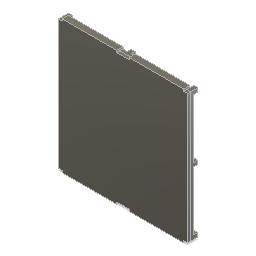
LED Cover v2 (Autodesk Fusion 360 design; units mm, degrees)
Autodesk Fusion 360 part; units mm, degrees
(part 1 of 3)
sketch "Skizze1" plane through (0, 0, 0) normal (0, 0, 1) x (1, 0, 0)
  line L0 (0, 0) -> (161, 0)
  line L1 (161, 0) -> (161, 161)
  line L2 (161, 161) -> (0, 161)
  line L3 (0, 161) -> (0, 0)
  line L4 (0, 0) -> (-2.4, 0) construction
  line L5 (-2.4, 0) -> (-2.4, -2.4) construction
  line L6 (-2.4, -2.4) -> (0, -2.4) construction
  line L7 (0, -2.4) -> (0, 0) construction
  line L8 (-2.4, -2.4) -> (163.4, -2.4)
  line L9 (163.4, -2.4) -> (163.4, 163.4)
  line L10 (163.4, 163.4) -> (-2.4, 163.4)
  line L11 (-2.4, 163.4) -> (-2.4, -2.4)
  dimension "d1" = 161
  dimension "d2" = 161
  dimension "d3" = 2.4
  dimension "d5" = 2.4
  dimension "d6" = 165.8
  dimension "d7" = 165.8
  constraint horizontal L0
  constraint vertical L1
  constraint horizontal L2
  constraint vertical L3
  constraint coincident L0.start L3.end
  constraint horizontal L4
  constraint vertical L5
  constraint horizontal L6
  constraint vertical L7
  constraint horizontal L8
  constraint vertical L9
  constraint horizontal L10
  constraint vertical L11
  measures "d1" distance of L0.start L0.end
  measures "d2" distance of L0.start L2.end
  measures "d3" distance of L5.end L6.end
  measures "d5" distance of L4.end L5.end
  measures "d6" distance of L5.end L8.end
  measures "d7" distance of L5.end L10.end
extrude "Extrusion1" add sketch "Skizze1" against normal blind 4 contours L0 L1 L2 L3 | L8 L9 L10 L11 makes body 1
sketch "Skizze2" plane through (0, 0, -4) normal (0, 0, -1) x (-1, 0, 0)
  line L0 (2.4, -2.4) -> (2.4, 163.4)
  line L1 (2.4, 163.4) -> (-163.4, 163.4)
  line L2 (-163.4, 163.4) -> (-163.4, -2.4)
  line L3 (-163.4, -2.4) -> (2.4, -2.4)
  line L4 (2.4, 163.4) -> (0, 163.4) construction
  line L5 (0, 163.4) -> (0, 161) construction
  line L6 (0, 161) -> (2.4, 161) construction
  line L7 (2.4, 161) -> (2.4, 163.4) construction
  line L8 (0, 161) -> (-35, 161) construction
  line L9 (-35, 161) -> (-35, 131) construction
  line L10 (-35, 131) -> (-35, 111) construction
  line L11 (-35, 111) -> (-35, 91) construction
  line L12 (-35, 91) -> (-35, 71) construction
  line L13 (-35, 71) -> (-35, 51) construction
  line L14 (-35, 51) -> (-35, 31) construction
  circle A0 centre (-35, 121) radius 10
  circle A1 centre (-35, 81) radius 10
  circle A2 centre (-35, 41) radius 10
  line L15 (-25, 121) -> (2.4, 121) construction
  line L16 (2.4, 121) -> (2.4, 116)
  line L17 (2.4, 116) -> (-26.3397, 116)
  line L18 (2.4, 121) -> (2.4, 126) construction
  line L19 (2.4, 126) -> (-26.3397, 126)
  line L20 (2.4, 81) -> (2.4, 76)
  line L21 (2.4, 76) -> (-26.3397, 76)
  line L22 (2.4, 81) -> (2.4, 86)
  line L23 (2.4, 86) -> (-26.3397, 86)
  line L24 (2.4, 41) -> (2.4, 36)
  line L25 (2.4, 36) -> (-26.3397, 36)
  line L26 (2.4, 41) -> (2.4, 46)
  line L27 (2.4, 46) -> (-26.3397, 46)
  line L28 (-25, 121) -> (-35, 121) construction
  line L29 (-35, 31) -> (2.4, 31) construction
  line L30 (-35, 51) -> (2.4, 51) construction
  line L31 (-35, 71) -> (2.4, 71) construction
  line L32 (-35, 91) -> (2.4, 91) construction
  line L33 (-35, 111) -> (2.4, 111) construction
  line L34 (-35, 131) -> (2.4, 131) construction
  line L35 (2.4, 131) -> (-2.6, 131)
  line L36 (-2.6, 131) -> (-2.6, 111)
  line L37 (-2.6, 111) -> (2.4, 111)
  line L38 (2.4, 111) -> (2.4, 131)
  line L39 (2.4, 91) -> (-2.6, 91)
  line L40 (-2.6, 91) -> (-2.6, 71)
  line L41 (-2.6, 71) -> (2.4, 71)
  line L42 (2.4, 71) -> (2.4, 91)
  line L43 (2.4, 51) -> (-2.6, 51)
  line L44 (-2.6, 51) -> (-2.6, 31)
  line L45 (-2.6, 31) -> (2.4, 31)
  line L46 (2.4, 31) -> (2.4, 51)
  line L47 (2.4, -2.4) -> (-2.6, -2.4)
  line L48 (-2.6, -2.4) -> (-2.6, 2.6)
  line L49 (-2.6, 2.6) -> (2.4, 2.6)
  line L50 (2.4, 2.6) -> (2.4, -2.4)
  line L51 (-78, 2.6) -> (-78, -2.4)
  line L52 (-78, -2.4) -> (-83, -2.4)
  line L53 (-83, 2.6) -> (-78, 2.6)
  line L54 (-83, -2.4) -> (-83, 2.6)
  line L55 (-158.4, 2.6) -> (-158.4, -2.4)
  line L56 (-158.4, -2.4) -> (-163.4, -2.4)
  line L57 (-163.4, 2.6) -> (-158.4, 2.6)
  line L58 (-163.4, -2.4) -> (-163.4, 2.6)
  line L59 (2.4, 83) -> (2.4, 78)
  line L60 (2.4, 78) -> (-2.6, 78)
  line L61 (-2.6, 83) -> (2.4, 83)
  line L62 (-2.6, 78) -> (-2.6, 83)
  line L63 (-78, 83) -> (-78, 78)
  line L64 (-78, 78) -> (-83, 78)
  line L65 (-83, 83) -> (-78, 83)
  line L66 (-83, 78) -> (-83, 83)
  line L67 (-158.4, 83) -> (-158.4, 78)
  line L68 (-158.4, 78) -> (-163.4, 78)
  line L69 (-163.4, 83) -> (-158.4, 83)
  line L70 (-163.4, 78) -> (-163.4, 83)
  line L71 (2.4, 163.4) -> (2.4, 158.4)
  line L72 (2.4, 158.4) -> (-2.6, 158.4)
  line L73 (-2.6, 163.4) -> (2.4, 163.4)
  line L74 (-2.6, 158.4) -> (-2.6, 163.4)
  line L75 (-78, 163.4) -> (-78, 158.4)
  line L76 (-78, 158.4) -> (-83, 158.4)
  line L77 (-83, 163.4) -> (-78, 163.4)
  line L78 (-83, 158.4) -> (-83, 163.4)
  line L79 (-158.4, 163.4) -> (-158.4, 158.4)
  line L80 (-158.4, 158.4) -> (-163.4, 158.4)
  line L81 (-163.4, 163.4) -> (-158.4, 163.4)
  line L82 (-163.4, 158.4) -> (-163.4, 163.4)
  circle A3 centre (-35, 121) radius 10.9
  line L83 (-26.3397, 126) -> (-26.3397, 127.8) construction
  line L84 (-26.3397, 127.8) -> (-2.6, 127.8)
  line L85 (-26.3397, 127.8) -> (-27.6679, 127.8)
  line L86 (-26.3397, 114.2) -> (-27.6679, 114.2)
  line L87 (-26.3397, 114.2) -> (-2.6, 114.2)
  line L88 (-26.3397, 74.2) -> (-2.6, 74.2)
  line L89 (-26.3397, 74.2) -> (-27.6679, 74.2)
  line L90 (-26.3397, 87.8) -> (-27.6679, 87.8)
  line L91 (-26.3397, 87.8) -> (-2.6, 87.8)
  circle A4 centre (-35, 81) radius 10.9
  line L92 (-26.3397, 34.2) -> (-2.6, 34.2)
  line L93 (-26.3397, 34.2) -> (-27.6679, 34.2)
  line L94 (-26.3397, 47.8) -> (-27.6679, 47.8)
  line L95 (-26.3397, 47.8) -> (-2.6, 47.8)
  circle A5 centre (-35, 41) radius 10.9
  dimension "d12" = 2.4
  dimension "d13" = 2.4
  dimension "d14" = 35
  dimension "d15" = 30
  dimension "d16" = 20
  dimension "d17" = 20
  dimension "d18" = 20
  dimension "d19" = 20
  dimension "d20" = 20
  dimension "d21" = 20
  dimension "d22" = 20
  dimension "d23" = 20
  dimension "d24" = 5
  dimension "d27" = 0
  dimension "d28" = -80
  dimension "d31" = 5
  dimension "d32" = 5
  dimension "d33" = 5
  dimension "d34" = 5
  dimension "d35" = 5
  dimension "d38" = -160.8
  dimension "d39" = 160.8
  dimension "d74" = 21.8
  dimension "d75" = 1.8
  constraint horizontal L4
  constraint vertical L5
  constraint horizontal L6
  constraint vertical L7
  constraint coincident L0.end L1.start
  constraint perpendicular L5 L8
  constraint perpendicular L8 L9
  constraint parallel L9 L10
  constraint parallel L10 L11
  constraint parallel L11 L12
  constraint parallel L12 L13
  constraint parallel L13 L14
  constraint midpoint L10 A0.centre
  constraint midpoint L12 A1.centre
  constraint coincident L14 A2.centre
  constraint coincident A0 L15.start
  constraint coincident L0 L15.end
  constraint perpendicular L0 L15
  constraint perpendicular L15 L16
  constraint horizontal L17
  constraint coincident A0 L17.end
  constraint symmetric L16.start L15 L18.start
  constraint symmetric L15 L16.end L18.end
  constraint symmetric L15 L17.end L19.end
  constraint midpoint L14 A2.centre
  constraint coincident A0.centre L28.end
  constraint perpendicular L10 L28
  constraint coincident L0 L29.end
  constraint tangent A2 L29
  constraint perpendicular L0 L29
  constraint coincident L0 L30.end
  constraint tangent A2 L30
  constraint perpendicular L0 L30
  constraint coincident L0 L31.end
  constraint tangent A1 L31
  constraint perpendicular L0 L31
  constraint coincident L0 L32.end
  constraint tangent A1 L32
  constraint perpendicular L0 L32
  constraint coincident L0 L33.end
  constraint tangent A0 L33
  constraint perpendicular L0 L33
  constraint coincident L0 L34.end
  constraint tangent A0 L34
  constraint perpendicular L0 L34
  constraint horizontal L35
  constraint vertical L36
  constraint horizontal L37
  constraint vertical L38
  constraint horizontal L39
  constraint vertical L40
  constraint horizontal L41
  constraint vertical L42
  constraint coincident L31 L40.end
  constraint horizontal L43
  constraint vertical L44
  constraint horizontal L45
  constraint vertical L46
  constraint coincident L29 L44.end
  constraint horizontal L47
  constraint vertical L48
  constraint horizontal L49
  constraint vertical L50
  constraint coincident L0.start L3.end
  constraint vertical L83
  constraint horizontal L84
  constraint coincident L36 L84.end
  constraint coincident A0 L85.end
  constraint perpendicular L83 L85
  constraint symmetric L15 L83.end L86.start
  constraint symmetric L15 L84.end L87.end
  constraint symmetric L15 L85.end L86.end
  measures "d12" distance of L0.end L4.end
  measures "d13" distance of L0.end L6.end
  measures "d14" distance of L5.end L8.end
  measures "d15" distance of L8.end L9.end
  measures "d16" distance of L9.end L10.end
  measures "d17" distance of L10.end L11.end
  measures "d18" distance of L11.end L12.end
  measures "d19" distance of L12.end L13.end
  measures "d20" distance of L13.end L14.end
  measures "d24" distance of L15.end L16.end
  measures "d31" distance of L34.end L35.end
  measures "d32" distance of L32.end L39.end
  measures "d33" distance of L30.end L43.end
  measures "d34" distance of L0.start L47.end
  measures "d35" distance of L0.start L49.end
  measures "d75" distance of L19.end L83.end
extrude "Extrusion3" cut sketch "Skizze2" against normal blind 5 contours L0 L24 L25 L26 L27 L44 L46 | L25 L27 L44 A5 | A2 L25 L27 A5 | A2 | L0 L20 L21 L40 L42 L60 | L0 L20 L22 L40 L42 L59 L60 L61 L62 | L21 L23 L40 L62 A4 | A1 L21 L23 A4 | L0 L22 L23 L40 L42 L61 | A1 | L0 L16 L17 L19 L36 L38 | L17 L19 L36 A3 | A0 L17 L19 A3 | A0 bodies 1
extrude "Extrusion4" add sketch "Skizze2" along normal blind 5 contours L0 L3 L47 L48 L49 L50 | L3 L51 L52 L53 L54 | L2 L3 L55 L56 L57 L58 | L2 L67 L68 L69 L70 | L0 L20 L22 L40 L42 L59 L60 L61 L62 | L1 L2 L79 L80 L81 L82 | L1 L75 L76 L77 L78 | L0 L1 L71 L72 L73 L74 | L63 L64 L65 L66 bodies 1 makes body 2 at (-0.7333, 78, -5.6667)
extrude "Extrusion9" add sketch "Skizze2" along normal blind 1 contours L0 L25 L44 L45 L46 | L0 L24 L25 L26 L27 L44 L46 | L25 L44 L92 L93 A5 | L25 L27 L44 A5 | L0 L27 L43 L44 L46 | A2 L25 L93 A5 | A2 L25 L27 A5 | L27 L44 L94 L95 A5 | A2 | A2 L93 L94 A5 | A2 L27 L94 A5 | L0 L21 L40 L41 L42 | L0 L20 L21 L40 L42 L60 | L0 L20 L22 L40 L42 L59 L60 L61 L62 | L21 L40 L88 L89 A4 | L21 L23 L40 L62 A4 | A1 L21 L89 A4 | A1 L21 L23 A4 | L0 L22 L23 L40 L42 L61 | A1 | A1 L89 L90 A4 | L0 L23 L39 L40 L42 | L23 L40 L90 L91 A4 | A1 L23 L90 A4 | L0 L17 L36 L37 L38 | L0 L16 L17 L19 L36 L38 | L17 L36 A3 L86 L87 | L17 L19 L36 A3 | L0 L19 L35 L36 L38 | A0 L17 A3 L86 | A0 L17 L19 A3 | L19 L36 A3 L84 L85 | A0 | A0 A3 L85 L86 | A0 L19 A3 L85 bodies 2 1
sketch "Skizze3" plane through (0, 0, 0) normal (0, 0, 1) x (1, 0, 0)
  line L0 (-2.4, 86) -> (26.3397, 86)
  arc A0 (26.3397, 76) -> (26.3397, 86) centre (35, 81) ccw
  line L1 (26.3397, 76) -> (-2.4, 76)
  line L2 (-2.4, 76) -> (-2.4, 46)
  line L3 (-2.4, 46) -> (26.3397, 46)
  arc A1 (26.3397, 36) -> (26.3397, 46) centre (35, 41) ccw
  line L4 (26.3397, 36) -> (-2.4, 36)
  line L5 (-2.4, 36) -> (-2.4, -2.4)
  line L6 (-2.4, -2.4) -> (163.4, -2.4)
  line L7 (163.4, -2.4) -> (163.4, 163.4)
  line L8 (163.4, 163.4) -> (-2.4, 163.4)
  line L9 (-2.4, 163.4) -> (-2.4, 126)
  line L10 (-2.4, 126) -> (26.3397, 126)
  arc A2 (26.3397, 116) -> (26.3397, 126) centre (35, 121) ccw
  line L11 (26.3397, 116) -> (-2.4, 116)
  line L12 (-2.4, 116) -> (-2.4, 86)
  line L13 (163.4, 163.4) -> (-2.4, 163.4)
  line L14 (-2.4, 163.4) -> (-2.4, -2.4)
  line L15 (-2.4, -2.4) -> (163.4, -2.4)
  line L16 (163.4, -2.4) -> (163.4, 163.4)
  line L17 (-2.4, -2.4) -> (0, -2.4) construction
  line L18 (0, -2.4) -> (0, 0) construction
  line L19 (0, 0) -> (-2.4, 0) construction
  line L20 (-2.4, 0) -> (-2.4, -2.4) construction
  line L21 (0, 0) -> (161, 0)
  line L22 (161, 0) -> (161, 161)
  line L23 (161, 161) -> (0, 161)
  line L24 (0, 161) -> (0, 0)
  line L25 (-2.4, 163.4) -> (72.6, 163.4)
  line L26 (72.6, 163.4) -> (72.6, 165.9)
  line L27 (72.6, 165.9) -> (-2.4, 165.9)
  line L28 (-2.4, 165.9) -> (-2.4, 163.4)
  line L29 (-2.4, 165.9) -> (2.6, 165.9) construction
  line L30 (2.6, 165.9) -> (2.6, 163.4)
  line L31 (2.6, 163.4) -> (2.6, 161)
  line L32 (80.5, 161) -> (80.5, 144.4743) construction
  line L33 (161, 80.5) -> (141.9366, 80.5) construction
  line L34 (163.4, 163.4) -> (88.4, 163.4)
  line L35 (88.4, 163.4) -> (88.4, 165.9)
  line L36 (88.4, 165.9) -> (163.4, 165.9)
  line L37 (163.4, 165.9) -> (163.4, 163.4)
  line L38 (158.4, 163.4) -> (158.4, 161)
  line L39 (158.4, 165.9) -> (158.4, 163.4)
  line L40 (163.4, -2.4) -> (88.4, -2.4)
  line L41 (88.4, -2.4) -> (88.4, -4.9)
  line L42 (88.4, -4.9) -> (163.4, -4.9)
  line L43 (163.4, -4.9) -> (163.4, -2.4)
  line L44 (158.4, -2.4) -> (158.4, 0)
  line L45 (158.4, -4.9) -> (158.4, -2.4)
  line L46 (-2.4, -2.4) -> (72.6, -2.4)
  line L47 (72.6, -2.4) -> (72.6, -4.9)
  line L48 (-2.4, -4.9) -> (-2.4, -2.4)
  line L49 (2.6, -2.4) -> (2.6, 0)
  line L50 (2.6, -4.9) -> (2.6, -2.4)
  line L51 (72.6, -4.9) -> (-2.4, -4.9)
  line L52 (88.4, 163.4) -> (88.4, 161)
  line L53 (72.6, 163.4) -> (72.6, 161)
  line L54 (72.6, -2.4) -> (72.6, 0)
  line L55 (88.4, -2.4) -> (88.4, 0)
  dimension "d42" = 2.4
  dimension "d43" = 2.4
  dimension "d44" = 161
  dimension "d45" = 161
  dimension "d46" = 75
  dimension "d47" = 2.5
  dimension "d48" = 5
  constraint horizontal L13
  constraint vertical L14
  constraint horizontal L15
  constraint vertical L16
  constraint coincident L5.end L6.start
  constraint coincident L7.end L8.start
  constraint horizontal L17
  constraint vertical L18
  constraint horizontal L19
  constraint vertical L20
  constraint horizontal L21
  constraint vertical L22
  constraint horizontal L23
  constraint vertical L24
  constraint coincident L18.end L19.start
  constraint horizontal L25
  constraint vertical L26
  constraint horizontal L27
  constraint vertical L28
  constraint coincident L8.end L9.start
  constraint perpendicular L28 L29
  constraint vertical L30
  constraint coincident L25 L30.end
  constraint coincident L23 L31.end
  constraint perpendicular L23 L31
  constraint midpoint L23 L32.start
  constraint perpendicular L23 L32
  constraint midpoint L22 L33.start
  constraint perpendicular L22 L33
  constraint symmetric L8.end L32 L7.end
  constraint symmetric L25.end L32 L34.end
  constraint symmetric L26.end L32 L35.end
  constraint symmetric L27.end L32 L36.end
  constraint symmetric L29.end L32 L39.start
  constraint symmetric L30.end L32 L38.start
  constraint symmetric L31.end L32 L38.end
  constraint symmetric L8.end L33 L5.end
  constraint symmetric L25.end L33 L46.end
  constraint symmetric L26.end L33 L47.end
  constraint symmetric L27.end L33 L48.start
  constraint symmetric L29.end L33 L50.start
  constraint symmetric L30.end L33 L49.start
  constraint symmetric L31.end L33 L49.end
  constraint symmetric L33 L7.end L6.end
  constraint symmetric L33 L34.end L40.end
  constraint symmetric L33 L35.end L41.end
  constraint symmetric L33 L36.end L42.end
  constraint symmetric L33 L38.start L44.start
  constraint symmetric L33 L38.end L44.end
  constraint symmetric L33 L39.start L45.start
  constraint coincident L23 L52.end
  constraint perpendicular L23 L52
  constraint symmetric L32 L34.end L25.end
  constraint symmetric L32 L52.end L53.end
  constraint symmetric L33 L52.end L55.end
  constraint symmetric L33 L25.end L46.end
  constraint symmetric L33 L53.end L54.end
  measures "d42" distance of L5.end L17.end
  measures "d43" distance of L5.end L19.end
  measures "d44" distance of L18.end L21.end
  measures "d45" distance of L18.end L23.end
  measures "d46" distance of L8.end L25.end
  measures "d47" distance of L8.end L27.end
  measures "d48" distance of L27.end L29.end
extrude "Extrusion5" add sketch "Skizze3" along normal blind 2 separate body contours L0 L11 L12 L14 L24 | L0 L1 L14 L24 | L10 L11 L14 L24 | L1 L2 L3 L14 L24 | L8 L9 L10 L13 L14 L23 L24 L25 L31 | L3 L4 L14 L24 | L4 L5 L6 L14 L15 L21 L24 L46 L49 | L8 L13 L23 L25 L31 L53 | L8 L13 L23 L52 L53 | L6 L15 L21 L46 L49 L54 | L8 L13 L23 L34 L38 L52 | L6 L15 L21 L54 L55 | L6 L7 L8 L13 L15 L16 L21 L22 L23 L34 L38 L40 L44 | L6 L15 L21 L40 L44 L55 makes body 3
extrude "Extrusion6" add sketch "Skizze3" along normal blind 2 from surface at 2 contours L0 L11 L12 L14 L24 | L0 L1 L14 L24 | L0 A0 L1 L3 A1 L4 L10 A2 L11 L21 L22 L23 L24 | L0 A0 L1 L24 | L10 L11 L14 L24 | L1 L2 L3 L14 L24 | L10 A2 L11 L24 | L8 L9 L10 L13 L14 L23 L24 L25 L31 | L3 L4 L14 L24 | L3 A1 L4 L24 | L4 L5 L6 L14 L15 L21 L24 L46 L49 | L8 L13 L23 L25 L31 L53 | L8 L13 L23 L52 L53 | L6 L15 L21 L46 L49 L54 | L8 L13 L23 L34 L38 L52 | L6 L15 L21 L54 L55 | L6 L7 L8 L13 L15 L16 L21 L22 L23 L34 L38 L40 L44 | L6 L15 L21 L40 L44 L55 bodies 3
extrude "Extrusion7" add sketch "Skizze3" along normal up to surface (4 mm away) and the other way up to surface (4 mm away) contours L8 L13 L25 L26 L27 L30 | L6 L15 L46 L47 L50 L51 | L8 L13 L34 L35 L36 L39 | L6 L15 L40 L41 L42 L45 bodies 3
sketch "Skizze4" plane through (0, 0, 2) normal (0, 0, -1) x (-1, 0, 0)
  line L0 (-161, 0) -> (0, 0)
  line L1 (0, 0) -> (0, 161)
  line L2 (0, 161) -> (-161, 161)
  line L3 (-161, 161) -> (-161, 0)
  line L4 (0, 161) -> (-2.4, 161) construction
  line L5 (-2.4, 161) -> (-2.4, 158.6) construction
  line L6 (-2.4, 158.6) -> (0, 158.6) construction
  line L7 (0, 158.6) -> (0, 161) construction
  line L8 (-2.4, 158.6) -> (-158.6, 158.6) construction
  line L9 (-2.4, 158.6) -> (-2.4, 2.4) construction
  line L10 (-2.4, 158.6) -> (-11.4, 158.6)
  line L11 (-11.4, 158.6) -> (-11.4, 152.1)
  line L12 (-11.4, 152.1) -> (-2.4, 152.1)
  line L13 (-2.4, 152.1) -> (-2.4, 158.6)
  line L14 (-2.4, 158.6) -> (-3, 158.6) construction
  line L15 (-3, 158.6) -> (-3, 158) construction
  line L16 (-3, 158) -> (-2.4, 158) construction
  line L17 (-2.4, 158) -> (-2.4, 158.6) construction
  line L18 (-3, 158) -> (-10.8, 158)
  line L19 (-10.8, 158) -> (-10.8, 152.7)
  line L20 (-10.8, 152.7) -> (-3, 152.7)
  line L21 (-3, 152.7) -> (-3, 158)
  line L22 (-20.6533, 152.7) -> (-12.8533, 152.7)
  line L23 (-12.2533, 158.6) -> (-21.2533, 158.6)
  line L24 (-21.2533, 158.6) -> (-21.2533, 152.1)
  line L25 (-12.2533, 152.1) -> (-12.2533, 158.6)
  line L26 (-21.2533, 152.1) -> (-12.2533, 152.1)
  line L27 (-20.6533, 158) -> (-20.6533, 152.7)
  line L28 (-12.8533, 158) -> (-20.6533, 158)
  line L29 (-12.8533, 152.7) -> (-12.8533, 158)
  line L30 (-30.5067, 152.7) -> (-22.7067, 152.7)
  line L31 (-22.1067, 158.6) -> (-31.1067, 158.6)
  line L32 (-31.1067, 158.6) -> (-31.1067, 152.1)
  line L33 (-22.1067, 152.1) -> (-22.1067, 158.6)
  line L34 (-31.1067, 152.1) -> (-22.1067, 152.1)
  line L35 (-30.5067, 158) -> (-30.5067, 152.7)
  line L36 (-22.7067, 158) -> (-30.5067, 158)
  line L37 (-22.7067, 152.7) -> (-22.7067, 158)
  line L38 (-40.36, 152.7) -> (-32.56, 152.7)
  line L39 (-31.96, 158.6) -> (-40.96, 158.6)
  line L40 (-40.96, 158.6) -> (-40.96, 152.1)
  line L41 (-31.96, 152.1) -> (-31.96, 158.6)
  line L42 (-40.96, 152.1) -> (-31.96, 152.1)
  line L43 (-40.36, 158) -> (-40.36, 152.7)
  line L44 (-32.56, 158) -> (-40.36, 158)
  line L45 (-32.56, 152.7) -> (-32.56, 158)
  line L46 (-50.2133, 152.7) -> (-42.4133, 152.7)
  line L47 (-41.8133, 158.6) -> (-50.8133, 158.6)
  line L48 (-50.8133, 158.6) -> (-50.8133, 152.1)
  line L49 (-41.8133, 152.1) -> (-41.8133, 158.6)
  line L50 (-50.8133, 152.1) -> (-41.8133, 152.1)
  line L51 (-50.2133, 158) -> (-50.2133, 152.7)
  line L52 (-42.4133, 158) -> (-50.2133, 158)
  line L53 (-42.4133, 152.7) -> (-42.4133, 158)
  line L54 (-60.0667, 152.7) -> (-52.2667, 152.7)
  line L55 (-51.6667, 158.6) -> (-60.6667, 158.6)
  line L56 (-60.6667, 158.6) -> (-60.6667, 152.1)
  line L57 (-51.6667, 152.1) -> (-51.6667, 158.6)
  line L58 (-60.6667, 152.1) -> (-51.6667, 152.1)
  line L59 (-60.0667, 158) -> (-60.0667, 152.7)
  line L60 (-52.2667, 158) -> (-60.0667, 158)
  line L61 (-52.2667, 152.7) -> (-52.2667, 158)
  line L62 (-69.92, 152.7) -> (-62.12, 152.7)
  line L63 (-61.52, 158.6) -> (-70.52, 158.6)
  line L64 (-70.52, 158.6) -> (-70.52, 152.1)
  line L65 (-61.52, 152.1) -> (-61.52, 158.6)
  line L66 (-70.52, 152.1) -> (-61.52, 152.1)
  line L67 (-69.92, 158) -> (-69.92, 152.7)
  line L68 (-62.12, 158) -> (-69.92, 158)
  line L69 (-62.12, 152.7) -> (-62.12, 158)
  line L70 (-79.7733, 152.7) -> (-71.9733, 152.7)
  line L71 (-71.3733, 158.6) -> (-80.3733, 158.6)
  line L72 (-80.3733, 158.6) -> (-80.3733, 152.1)
  line L73 (-71.3733, 152.1) -> (-71.3733, 158.6)
  line L74 (-80.3733, 152.1) -> (-71.3733, 152.1)
  line L75 (-79.7733, 158) -> (-79.7733, 152.7)
  line L76 (-71.9733, 158) -> (-79.7733, 158)
  line L77 (-71.9733, 152.7) -> (-71.9733, 158)
  line L78 (-89.6267, 152.7) -> (-81.8267, 152.7)
  line L79 (-81.2267, 158.6) -> (-90.2267, 158.6)
  line L80 (-90.2267, 158.6) -> (-90.2267, 152.1)
  line L81 (-81.2267, 152.1) -> (-81.2267, 158.6)
  line L82 (-90.2267, 152.1) -> (-81.2267, 152.1)
  line L83 (-89.6267, 158) -> (-89.6267, 152.7)
  line L84 (-81.8267, 158) -> (-89.6267, 158)
  line L85 (-81.8267, 152.7) -> (-81.8267, 158)
  line L86 (-99.48, 152.7) -> (-91.68, 152.7)
  line L87 (-91.08, 158.6) -> (-100.08, 158.6)
  line L88 (-100.08, 158.6) -> (-100.08, 152.1)
  line L89 (-91.08, 152.1) -> (-91.08, 158.6)
  line L90 (-100.08, 152.1) -> (-91.08, 152.1)
  line L91 (-99.48, 158) -> (-99.48, 152.7)
  line L92 (-91.68, 158) -> (-99.48, 158)
  line L93 (-91.68, 152.7) -> (-91.68, 158)
  line L94 (-109.3333, 152.7) -> (-101.5333, 152.7)
  line L95 (-100.9333, 158.6) -> (-109.9333, 158.6)
  line L96 (-109.9333, 158.6) -> (-109.9333, 152.1)
  line L97 (-100.9333, 152.1) -> (-100.9333, 158.6)
  line L98 (-109.9333, 152.1) -> (-100.9333, 152.1)
  line L99 (-109.3333, 158) -> (-109.3333, 152.7)
  line L100 (-101.5333, 158) -> (-109.3333, 158)
  line L101 (-101.5333, 152.7) -> (-101.5333, 158)
  line L102 (-119.1867, 152.7) -> (-111.3867, 152.7)
  line L103 (-110.7867, 158.6) -> (-119.7867, 158.6)
  line L104 (-119.7867, 158.6) -> (-119.7867, 152.1)
  line L105 (-110.7867, 152.1) -> (-110.7867, 158.6)
  line L106 (-119.7867, 152.1) -> (-110.7867, 152.1)
  line L107 (-119.1867, 158) -> (-119.1867, 152.7)
  line L108 (-111.3867, 158) -> (-119.1867, 158)
  line L109 (-111.3867, 152.7) -> (-111.3867, 158)
  line L110 (-129.04, 152.7) -> (-121.24, 152.7)
  line L111 (-120.64, 158.6) -> (-129.64, 158.6)
  line L112 (-129.64, 158.6) -> (-129.64, 152.1)
  line L113 (-120.64, 152.1) -> (-120.64, 158.6)
  line L114 (-129.64, 152.1) -> (-120.64, 152.1)
  line L115 (-129.04, 158) -> (-129.04, 152.7)
  line L116 (-121.24, 158) -> (-129.04, 158)
  line L117 (-121.24, 152.7) -> (-121.24, 158)
  line L118 (-138.8933, 152.7) -> (-131.0933, 152.7)
  line L119 (-130.4933, 158.6) -> (-139.4933, 158.6)
  line L120 (-139.4933, 158.6) -> (-139.4933, 152.1)
  line L121 (-130.4933, 152.1) -> (-130.4933, 158.6)
  line L122 (-139.4933, 152.1) -> (-130.4933, 152.1)
  line L123 (-138.8933, 158) -> (-138.8933, 152.7)
  line L124 (-131.0933, 158) -> (-138.8933, 158)
  line L125 (-131.0933, 152.7) -> (-131.0933, 158)
  line L126 (-148.7467, 152.7) -> (-140.9467, 152.7)
  line L127 (-140.3467, 158.6) -> (-149.3467, 158.6)
  line L128 (-149.3467, 158.6) -> (-149.3467, 152.1)
  line L129 (-140.3467, 152.1) -> (-140.3467, 158.6)
  line L130 (-149.3467, 152.1) -> (-140.3467, 152.1)
  line L131 (-148.7467, 158) -> (-148.7467, 152.7)
  line L132 (-140.9467, 158) -> (-148.7467, 158)
  line L133 (-140.9467, 152.7) -> (-140.9467, 158)
  line L134 (-158.6, 152.7) -> (-150.8, 152.7)
  line L135 (-150.2, 158.6) -> (-159.2, 158.6)
  line L136 (-159.2, 158.6) -> (-159.2, 152.1)
  line L137 (-150.2, 152.1) -> (-150.2, 158.6)
  line L138 (-159.2, 152.1) -> (-150.2, 152.1)
  line L139 (-158.6, 158) -> (-158.6, 152.7)
  line L140 (-150.8, 158) -> (-158.6, 158)
  line L141 (-150.8, 152.7) -> (-150.8, 158)
  line L142 (-10.8, 142.68) -> (-3, 142.68)
  line L143 (-2.4, 148.58) -> (-11.4, 148.58)
  line L144 (-11.4, 148.58) -> (-11.4, 142.08)
  line L145 (-2.4, 142.08) -> (-2.4, 148.58)
  line L146 (-11.4, 142.08) -> (-2.4, 142.08)
  line L147 (-10.8, 147.98) -> (-10.8, 142.68)
  line L148 (-3, 147.98) -> (-10.8, 147.98)
  line L149 (-3, 142.68) -> (-3, 147.98)
  line L150 (-20.6533, 142.68) -> (-12.8533, 142.68)
  line L151 (-12.2533, 148.58) -> (-21.2533, 148.58)
  line L152 (-21.2533, 148.58) -> (-21.2533, 142.08)
  line L153 (-12.2533, 142.08) -> (-12.2533, 148.58)
  line L154 (-21.2533, 142.08) -> (-12.2533, 142.08)
  line L155 (-20.6533, 147.98) -> (-20.6533, 142.68)
  line L156 (-12.8533, 147.98) -> (-20.6533, 147.98)
  line L157 (-12.8533, 142.68) -> (-12.8533, 147.98)
  line L158 (-30.5067, 142.68) -> (-22.7067, 142.68)
  line L159 (-22.1067, 148.58) -> (-31.1067, 148.58)
  line L160 (-31.1067, 148.58) -> (-31.1067, 142.08)
  line L161 (-22.1067, 142.08) -> (-22.1067, 148.58)
  line L162 (-31.1067, 142.08) -> (-22.1067, 142.08)
  line L163 (-30.5067, 147.98) -> (-30.5067, 142.68)
  line L164 (-22.7067, 147.98) -> (-30.5067, 147.98)
  line L165 (-22.7067, 142.68) -> (-22.7067, 147.98)
  line L166 (-40.36, 142.68) -> (-32.56, 142.68)
  line L167 (-31.96, 148.58) -> (-40.96, 148.58)
  line L168 (-40.96, 148.58) -> (-40.96, 142.08)
  line L169 (-31.96, 142.08) -> (-31.96, 148.58)
  line L170 (-40.96, 142.08) -> (-31.96, 142.08)
  line L171 (-40.36, 147.98) -> (-40.36, 142.68)
  line L172 (-32.56, 147.98) -> (-40.36, 147.98)
  line L173 (-32.56, 142.68) -> (-32.56, 147.98)
  line L174 (-50.2133, 142.68) -> (-42.4133, 142.68)
  line L175 (-41.8133, 148.58) -> (-50.8133, 148.58)
  line L176 (-50.8133, 148.58) -> (-50.8133, 142.08)
  line L177 (-41.8133, 142.08) -> (-41.8133, 148.58)
  line L178 (-50.8133, 142.08) -> (-41.8133, 142.08)
  line L179 (-50.2133, 147.98) -> (-50.2133, 142.68)
  line L180 (-42.4133, 147.98) -> (-50.2133, 147.98)
  line L181 (-42.4133, 142.68) -> (-42.4133, 147.98)
  line L182 (-60.0667, 142.68) -> (-52.2667, 142.68)
  line L183 (-51.6667, 148.58) -> (-60.6667, 148.58)
  line L184 (-60.6667, 148.58) -> (-60.6667, 142.08)
  line L185 (-51.6667, 142.08) -> (-51.6667, 148.58)
  line L186 (-60.6667, 142.08) -> (-51.6667, 142.08)
  line L187 (-60.0667, 147.98) -> (-60.0667, 142.68)
  line L188 (-52.2667, 147.98) -> (-60.0667, 147.98)
  line L189 (-52.2667, 142.68) -> (-52.2667, 147.98)
  line L190 (-69.92, 142.68) -> (-62.12, 142.68)
  line L191 (-61.52, 148.58) -> (-70.52, 148.58)
  line L192 (-70.52, 148.58) -> (-70.52, 142.08)
  line L193 (-61.52, 142.08) -> (-61.52, 148.58)
  line L194 (-70.52, 142.08) -> (-61.52, 142.08)
  line L195 (-69.92, 147.98) -> (-69.92, 142.68)
  line L196 (-62.12, 147.98) -> (-69.92, 147.98)
  line L197 (-62.12, 142.68) -> (-62.12, 147.98)
  line L198 (-79.7733, 142.68) -> (-71.9733, 142.68)
  line L199 (-71.3733, 148.58) -> (-80.3733, 148.58)
  line L200 (-80.3733, 148.58) -> (-80.3733, 142.08)
  line L201 (-71.3733, 142.08) -> (-71.3733, 148.58)
  line L202 (-80.3733, 142.08) -> (-71.3733, 142.08)
  line L203 (-79.7733, 147.98) -> (-79.7733, 142.68)
  line L204 (-71.9733, 147.98) -> (-79.7733, 147.98)
  line L205 (-71.9733, 142.68) -> (-71.9733, 147.98)
  line L206 (-89.6267, 142.68) -> (-81.8267, 142.68)
  line L207 (-81.2267, 148.58) -> (-90.2267, 148.58)
  line L208 (-90.2267, 148.58) -> (-90.2267, 142.08)
  line L209 (-81.2267, 142.08) -> (-81.2267, 148.58)
  line L210 (-90.2267, 142.08) -> (-81.2267, 142.08)
  line L211 (-89.6267, 147.98) -> (-89.6267, 142.68)
  line L212 (-81.8267, 147.98) -> (-89.6267, 147.98)
  line L213 (-81.8267, 142.68) -> (-81.8267, 147.98)
  line L214 (-99.48, 142.68) -> (-91.68, 142.68)
  line L215 (-91.08, 148.58) -> (-100.08, 148.58)
  line L216 (-100.08, 148.58) -> (-100.08, 142.08)
  line L217 (-91.08, 142.08) -> (-91.08, 148.58)
  line L218 (-100.08, 142.08) -> (-91.08, 142.08)
  line L219 (-99.48, 147.98) -> (-99.48, 142.68)
  line L220 (-91.68, 147.98) -> (-99.48, 147.98)
  line L221 (-91.68, 142.68) -> (-91.68, 147.98)
  line L222 (-109.3333, 142.68) -> (-101.5333, 142.68)
  line L223 (-100.9333, 148.58) -> (-109.9333, 148.58)
  line L224 (-109.9333, 148.58) -> (-109.9333, 142.08)
  line L225 (-100.9333, 142.08) -> (-100.9333, 148.58)
  line L226 (-109.9333, 142.08) -> (-100.9333, 142.08)
  line L227 (-109.3333, 147.98) -> (-109.3333, 142.68)
  line L228 (-101.5333, 147.98) -> (-109.3333, 147.98)
  line L229 (-101.5333, 142.68) -> (-101.5333, 147.98)
  line L230 (-119.1867, 142.68) -> (-111.3867, 142.68)
  line L231 (-110.7867, 148.58) -> (-119.7867, 148.58)
  line L232 (-119.7867, 148.58) -> (-119.7867, 142.08)
  line L233 (-110.7867, 142.08) -> (-110.7867, 148.58)
  line L234 (-119.7867, 142.08) -> (-110.7867, 142.08)
  line L235 (-119.1867, 147.98) -> (-119.1867, 142.68)
  line L236 (-111.3867, 147.98) -> (-119.1867, 147.98)
  line L237 (-111.3867, 142.68) -> (-111.3867, 147.98)
  line L238 (-129.04, 142.68) -> (-121.24, 142.68)
  line L239 (-120.64, 148.58) -> (-129.64, 148.58)
  line L240 (-129.64, 148.58) -> (-129.64, 142.08)
  line L241 (-120.64, 142.08) -> (-120.64, 148.58)
  line L242 (-129.64, 142.08) -> (-120.64, 142.08)
  line L243 (-129.04, 147.98) -> (-129.04, 142.68)
  line L244 (-121.24, 147.98) -> (-129.04, 147.98)
  line L245 (-121.24, 142.68) -> (-121.24, 147.98)
  line L246 (-138.8933, 142.68) -> (-131.0933, 142.68)
  line L247 (-130.4933, 148.58) -> (-139.4933, 148.58)
  line L248 (-139.4933, 148.58) -> (-139.4933, 142.08)
  line L249 (-130.4933, 142.08) -> (-130.4933, 148.58)
  line L250 (-139.4933, 142.08) -> (-130.4933, 142.08)
  line L251 (-138.8933, 147.98) -> (-138.8933, 142.68)
  line L252 (-131.0933, 147.98) -> (-138.8933, 147.98)
  line L253 (-131.0933, 142.68) -> (-131.0933, 147.98)
  line L254 (-148.7467, 142.68) -> (-140.9467, 142.68)
  line L255 (-140.3467, 148.58) -> (-149.3467, 148.58)
  line L256 (-149.3467, 148.58) -> (-149.3467, 142.08)
  line L257 (-140.3467, 142.08) -> (-140.3467, 148.58)
  line L258 (-149.3467, 142.08) -> (-140.3467, 142.08)
  line L259 (-148.7467, 147.98) -> (-148.7467, 142.68)
  line L260 (-140.9467, 147.98) -> (-148.7467, 147.98)
  line L261 (-140.9467, 142.68) -> (-140.9467, 147.98)
  line L262 (-158.6, 142.68) -> (-150.8, 142.68)
  line L263 (-150.2, 148.58) -> (-159.2, 148.58)
  line L264 (-159.2, 148.58) -> (-159.2, 142.08)
  line L265 (-150.2, 142.08) -> (-150.2, 148.58)
  line L266 (-159.2, 142.08) -> (-150.2, 142.08)
  line L267 (-158.6, 147.98) -> (-158.6, 142.68)
  line L268 (-150.8, 147.98) -> (-158.6, 147.98)
  line L269 (-150.8, 142.68) -> (-150.8, 147.98)
  line L270 (-10.8, 132.66) -> (-3, 132.66)
  line L271 (-2.4, 138.56) -> (-11.4, 138.56)
  line L272 (-11.4, 138.56) -> (-11.4, 132.06)
  line L273 (-2.4, 132.06) -> (-2.4, 138.56)
  line L274 (-11.4, 132.06) -> (-2.4, 132.06)
  line L275 (-10.8, 137.96) -> (-10.8, 132.66)
  line L276 (-3, 137.96) -> (-10.8, 137.96)
  line L277 (-3, 132.66) -> (-3, 137.96)
  line L278 (-20.6533, 132.66) -> (-12.8533, 132.66)
  line L279 (-12.2533, 138.56) -> (-21.2533, 138.56)
  line L280 (-21.2533, 138.56) -> (-21.2533, 132.06)
  line L281 (-12.2533, 132.06) -> (-12.2533, 138.56)
  line L282 (-21.2533, 132.06) -> (-12.2533, 132.06)
  line L283 (-20.6533, 137.96) -> (-20.6533, 132.66)
  line L284 (-12.8533, 137.96) -> (-20.6533, 137.96)
  line L285 (-12.8533, 132.66) -> (-12.8533, 137.96)
  line L286 (-30.5067, 132.66) -> (-22.7067, 132.66)
  line L287 (-22.1067, 138.56) -> (-31.1067, 138.56)
  line L288 (-31.1067, 138.56) -> (-31.1067, 132.06)
  line L289 (-22.1067, 132.06) -> (-22.1067, 138.56)
  line L290 (-31.1067, 132.06) -> (-22.1067, 132.06)
  line L291 (-30.5067, 137.96) -> (-30.5067, 132.66)
  line L292 (-22.7067, 137.96) -> (-30.5067, 137.96)
  line L293 (-22.7067, 132.66) -> (-22.7067, 137.96)
  line L294 (-40.36, 132.66) -> (-32.56, 132.66)
  line L295 (-31.96, 138.56) -> (-40.96, 138.56)
  line L296 (-40.96, 138.56) -> (-40.96, 132.06)
  line L297 (-31.96, 132.06) -> (-31.96, 138.56)
  line L298 (-40.96, 132.06) -> (-31.96, 132.06)
  line L299 (-40.36, 137.96) -> (-40.36, 132.66)
  line L300 (-32.56, 137.96) -> (-40.36, 137.96)
  line L301 (-32.56, 132.66) -> (-32.56, 137.96)
  line L302 (-50.2133, 132.66) -> (-42.4133, 132.66)
  line L303 (-41.8133, 138.56) -> (-50.8133, 138.56)
  line L304 (-50.8133, 138.56) -> (-50.8133, 132.06)
  line L305 (-41.8133, 132.06) -> (-41.8133, 138.56)
  line L306 (-50.8133, 132.06) -> (-41.8133, 132.06)
  line L307 (-50.2133, 137.96) -> (-50.2133, 132.66)
  line L308 (-42.4133, 137.96) -> (-50.2133, 137.96)
  line L309 (-42.4133, 132.66) -> (-42.4133, 137.96)
  line L310 (-60.0667, 132.66) -> (-52.2667, 132.66)
  line L311 (-51.6667, 138.56) -> (-60.6667, 138.56)
  line L312 (-60.6667, 138.56) -> (-60.6667, 132.06)
  line L313 (-51.6667, 132.06) -> (-51.6667, 138.56)
  line L314 (-60.6667, 132.06) -> (-51.6667, 132.06)
  line L315 (-60.0667, 137.96) -> (-60.0667, 132.66)
  line L316 (-52.2667, 137.96) -> (-60.0667, 137.96)
  line L317 (-52.2667, 132.66) -> (-52.2667, 137.96)
  line L318 (-69.92, 132.66) -> (-62.12, 132.66)
  line L319 (-61.52, 138.56) -> (-70.52, 138.56)
  line L320 (-70.52, 138.56) -> (-70.52, 132.06)
  line L321 (-61.52, 132.06) -> (-61.52, 138.56)
  line L322 (-70.52, 132.06) -> (-61.52, 132.06)
  line L323 (-69.92, 137.96) -> (-69.92, 132.66)
  line L324 (-62.12, 137.96) -> (-69.92, 137.96)
  line L325 (-62.12, 132.66) -> (-62.12, 137.96)
  line L326 (-79.7733, 132.66) -> (-71.9733, 132.66)
  line L327 (-71.3733, 138.56) -> (-80.3733, 138.56)
  line L328 (-80.3733, 138.56) -> (-80.3733, 132.06)
  line L329 (-71.3733, 132.06) -> (-71.3733, 138.56)
  line L330 (-80.3733, 132.06) -> (-71.3733, 132.06)
  line L331 (-79.7733, 137.96) -> (-79.7733, 132.66)
  line L332 (-71.9733, 137.96) -> (-79.7733, 137.96)
  line L333 (-71.9733, 132.66) -> (-71.9733, 137.96)
  line L334 (-89.6267, 132.66) -> (-81.8267, 132.66)
  line L335 (-81.2267, 138.56) -> (-90.2267, 138.56)
  line L336 (-90.2267, 138.56) -> (-90.2267, 132.06)
  line L337 (-81.2267, 132.06) -> (-81.2267, 138.56)
  line L338 (-90.2267, 132.06) -> (-81.2267, 132.06)
  line L339 (-89.6267, 137.96) -> (-89.6267, 132.66)
  line L340 (-81.8267, 137.96) -> (-89.6267, 137.96)
  line L341 (-81.8267, 132.66) -> (-81.8267, 137.96)
  line L342 (-99.48, 132.66) -> (-91.68, 132.66)
  line L343 (-91.08, 138.56) -> (-100.08, 138.56)
  line L344 (-100.08, 138.56) -> (-100.08, 132.06)
  line L345 (-91.08, 132.06) -> (-91.08, 138.56)
  line L346 (-100.08, 132.06) -> (-91.08, 132.06)
  line L347 (-99.48, 137.96) -> (-99.48, 132.66)
  line L348 (-91.68, 137.96) -> (-99.48, 137.96)
  line L349 (-91.68, 132.66) -> (-91.68, 137.96)
  line L350 (-109.3333, 132.66) -> (-101.5333, 132.66)
  line L351 (-100.9333, 138.56) -> (-109.9333, 138.56)
  line L352 (-109.9333, 138.56) -> (-109.9333, 132.06)
  line L353 (-100.9333, 132.06) -> (-100.9333, 138.56)
  line L354 (-109.9333, 132.06) -> (-100.9333, 132.06)
  line L355 (-109.3333, 137.96) -> (-109.3333, 132.66)
  line L356 (-101.5333, 137.96) -> (-109.3333, 137.96)
  line L357 (-101.5333, 132.66) -> (-101.5333, 137.96)
  line L358 (-119.1867, 132.66) -> (-111.3867, 132.66)
  line L359 (-110.7867, 138.56) -> (-119.7867, 138.56)
  line L360 (-119.7867, 138.56) -> (-119.7867, 132.06)
  line L361 (-110.7867, 132.06) -> (-110.7867, 138.56)
  line L362 (-119.7867, 132.06) -> (-110.7867, 132.06)
  line L363 (-119.1867, 137.96) -> (-119.1867, 132.66)
  line L364 (-111.3867, 137.96) -> (-119.1867, 137.96)
  line L365 (-111.3867, 132.66) -> (-111.3867, 137.96)
  line L366 (-129.04, 132.66) -> (-121.24, 132.66)
  line L367 (-120.64, 138.56) -> (-129.64, 138.56)
  line L368 (-129.64, 138.56) -> (-129.64, 132.06)
  line L369 (-120.64, 132.06) -> (-120.64, 138.56)
  line L370 (-129.64, 132.06) -> (-120.64, 132.06)
  line L371 (-129.04, 137.96) -> (-129.04, 132.66)
  line L372 (-121.24, 137.96) -> (-129.04, 137.96)
  line L373 (-121.24, 132.66) -> (-121.24, 137.96)
  line L374 (-138.8933, 132.66) -> (-131.0933, 132.66)
  line L375 (-130.4933, 138.56) -> (-139.4933, 138.56)
  line L376 (-139.4933, 138.56) -> (-139.4933, 132.06)
  line L377 (-130.4933, 132.06) -> (-130.4933, 138.56)
  line L378 (-139.4933, 132.06) -> (-130.4933, 132.06)
  line L379 (-138.8933, 137.96) -> (-138.8933, 132.66)
  line L380 (-131.0933, 137.96) -> (-138.8933, 137.96)
  line L381 (-131.0933, 132.66) -> (-131.0933, 137.96)
  line L382 (-148.7467, 132.66) -> (-140.9467, 132.66)
  line L383 (-140.3467, 138.56) -> (-149.3467, 138.56)
  line L384 (-149.3467, 138.56) -> (-149.3467, 132.06)
  line L385 (-140.3467, 132.06) -> (-140.3467, 138.56)
  line L386 (-149.3467, 132.06) -> (-140.3467, 132.06)
  line L387 (-148.7467, 137.96) -> (-148.7467, 132.66)
  line L388 (-140.9467, 137.96) -> (-148.7467, 137.96)
  line L389 (-140.9467, 132.66) -> (-140.9467, 137.96)
  line L390 (-158.6, 132.66) -> (-150.8, 132.66)
  line L391 (-150.2, 138.56) -> (-159.2, 138.56)
  line L392 (-159.2, 138.56) -> (-159.2, 132.06)
  line L393 (-150.2, 132.06) -> (-150.2, 138.56)
  line L394 (-159.2, 132.06) -> (-150.2, 132.06)
  line L395 (-158.6, 137.96) -> (-158.6, 132.66)
  line L396 (-150.8, 137.96) -> (-158.6, 137.96)
  line L397 (-150.8, 132.66) -> (-150.8, 137.96)
  line L398 (-10.8, 122.64) -> (-3, 122.64)
  line L399 (-2.4, 128.54) -> (-11.4, 128.54)
  line L400 (-11.4, 128.54) -> (-11.4, 122.04)
  line L401 (-2.4, 122.04) -> (-2.4, 128.54)
  line L402 (-11.4, 122.04) -> (-2.4, 122.04)
  line L403 (-10.8, 127.94) -> (-10.8, 122.64)
  line L404 (-3, 127.94) -> (-10.8, 127.94)
  line L405 (-3, 122.64) -> (-3, 127.94)
  line L406 (-20.6533, 122.64) -> (-12.8533, 122.64)
  line L407 (-12.2533, 128.54) -> (-21.2533, 128.54)
  line L408 (-21.2533, 128.54) -> (-21.2533, 122.04)
  line L409 (-12.2533, 122.04) -> (-12.2533, 128.54)
  line L410 (-21.2533, 122.04) -> (-12.2533, 122.04)
  line L411 (-20.6533, 127.94) -> (-20.6533, 122.64)
  line L412 (-12.8533, 127.94) -> (-20.6533, 127.94)
  line L413 (-12.8533, 122.64) -> (-12.8533, 127.94)
  line L414 (-30.5067, 122.64) -> (-22.7067, 122.64)
  line L415 (-22.1067, 128.54) -> (-31.1067, 128.54)
  line L416 (-31.1067, 128.54) -> (-31.1067, 122.04)
  line L417 (-22.1067, 122.04) -> (-22.1067, 128.54)
  line L418 (-31.1067, 122.04) -> (-22.1067, 122.04)
  line L419 (-30.5067, 127.94) -> (-30.5067, 122.64)
  line L420 (-22.7067, 127.94) -> (-30.5067, 127.94)
  line L421 (-22.7067, 122.64) -> (-22.7067, 127.94)
  line L422 (-40.36, 122.64) -> (-32.56, 122.64)
  line L423 (-31.96, 128.54) -> (-40.96, 128.54)
  line L424 (-40.96, 128.54) -> (-40.96, 122.04)
  line L425 (-31.96, 122.04) -> (-31.96, 128.54)
  line L426 (-40.96, 122.04) -> (-31.96, 122.04)
  line L427 (-40.36, 127.94) -> (-40.36, 122.64)
  line L428 (-32.56, 127.94) -> (-40.36, 127.94)
  line L429 (-32.56, 122.64) -> (-32.56, 127.94)
  line L430 (-50.2133, 122.64) -> (-42.4133, 122.64)
  line L431 (-41.8133, 128.54) -> (-50.8133, 128.54)
  line L432 (-50.8133, 128.54) -> (-50.8133, 122.04)
  line L433 (-41.8133, 122.04) -> (-41.8133, 128.54)
  line L434 (-50.8133, 122.04) -> (-41.8133, 122.04)
  line L435 (-50.2133, 127.94) -> (-50.2133, 122.64)
  line L436 (-42.4133, 127.94) -> (-50.2133, 127.94)
  line L437 (-42.4133, 122.64) -> (-42.4133, 127.94)
  line L438 (-60.0667, 122.64) -> (-52.2667, 122.64)
  line L439 (-51.6667, 128.54) -> (-60.6667, 128.54)
  line L440 (-60.6667, 128.54) -> (-60.6667, 122.04)
  line L441 (-51.6667, 122.04) -> (-51.6667, 128.54)
  line L442 (-60.6667, 122.04) -> (-51.6667, 122.04)
  line L443 (-60.0667, 127.94) -> (-60.0667, 122.64)
  line L444 (-52.2667, 127.94) -> (-60.0667, 127.94)
  line L445 (-52.2667, 122.64) -> (-52.2667, 127.94)
  line L446 (-69.92, 122.64) -> (-62.12, 122.64)
  line L447 (-61.52, 128.54) -> (-70.52, 128.54)
  line L448 (-70.52, 128.54) -> (-70.52, 122.04)
  line L449 (-61.52, 122.04) -> (-61.52, 128.54)
  line L450 (-70.52, 122.04) -> (-61.52, 122.04)
  line L451 (-69.92, 127.94) -> (-69.92, 122.64)
  line L452 (-62.12, 127.94) -> (-69.92, 127.94)
  line L453 (-62.12, 122.64) -> (-62.12, 127.94)
  line L454 (-79.7733, 122.64) -> (-71.9733, 122.64)
  line L455 (-71.3733, 128.54) -> (-80.3733, 128.54)
  line L456 (-80.3733, 128.54) -> (-80.3733, 122.04)
  line L457 (-71.3733, 122.04) -> (-71.3733, 128.54)
  line L458 (-80.3733, 122.04) -> (-71.3733, 122.04)
  line L459 (-79.7733, 127.94) -> (-79.7733, 122.64)
  line L460 (-71.9733, 127.94) -> (-79.7733, 127.94)
  line L461 (-71.9733, 122.64) -> (-71.9733, 127.94)
  line L462 (-89.6267, 122.64) -> (-81.8267, 122.64)
  line L463 (-81.2267, 128.54) -> (-90.2267, 128.54)
  line L464 (-90.2267, 128.54) -> (-90.2267, 122.04)
  line L465 (-81.2267, 122.04) -> (-81.2267, 128.54)
  line L466 (-90.2267, 122.04) -> (-81.2267, 122.04)
  line L467 (-89.6267, 127.94) -> (-89.6267, 122.64)
  line L468 (-81.8267, 127.94) -> (-89.6267, 127.94)
  line L469 (-81.8267, 122.64) -> (-81.8267, 127.94)
  line L470 (-99.48, 122.64) -> (-91.68, 122.64)
  line L471 (-91.08, 128.54) -> (-100.08, 128.54)
  line L472 (-100.08, 128.54) -> (-100.08, 122.04)
  line L473 (-91.08, 122.04) -> (-91.08, 128.54)
  line L474 (-100.08, 122.04) -> (-91.08, 122.04)
  line L475 (-99.48, 127.94) -> (-99.48, 122.64)
  line L476 (-91.68, 127.94) -> (-99.48, 127.94)
  line L477 (-91.68, 122.64) -> (-91.68, 127.94)
  line L478 (-109.3333, 122.64) -> (-101.5333, 122.64)
  line L479 (-100.9333, 128.54) -> (-109.9333, 128.54)
  line L480 (-109.9333, 128.54) -> (-109.9333, 122.04)
  line L481 (-100.9333, 122.04) -> (-100.9333, 128.54)
  line L482 (-109.9333, 122.04) -> (-100.9333, 122.04)
  line L483 (-109.3333, 127.94) -> (-109.3333, 122.64)
  line L484 (-101.5333, 127.94) -> (-109.3333, 127.94)
  line L485 (-101.5333, 122.64) -> (-101.5333, 127.94)
  line L486 (-119.1867, 122.64) -> (-111.3867, 122.64)
  line L487 (-110.7867, 128.54) -> (-119.7867, 128.54)
  line L488 (-119.7867, 128.54) -> (-119.7867, 122.04)
  line L489 (-110.7867, 122.04) -> (-110.7867, 128.54)
  line L490 (-119.7867, 122.04) -> (-110.7867, 122.04)
  line L491 (-119.1867, 127.94) -> (-119.1867, 122.64)
  line L492 (-111.3867, 127.94) -> (-119.1867, 127.94)
  line L493 (-111.3867, 122.64) -> (-111.3867, 127.94)
  line L494 (-129.04, 122.64) -> (-121.24, 122.64)
  line L495 (-120.64, 128.54) -> (-129.64, 128.54)
  line L496 (-129.64, 128.54) -> (-129.64, 122.04)
  line L497 (-120.64, 122.04) -> (-120.64, 128.54)
  line L498 (-129.64, 122.04) -> (-120.64, 122.04)
  line L499 (-129.04, 127.94) -> (-129.04, 122.64)
  line L500 (-121.24, 127.94) -> (-129.04, 127.94)
  line L501 (-121.24, 122.64) -> (-121.24, 127.94)
  line L502 (-138.8933, 122.64) -> (-131.0933, 122.64)
  line L503 (-130.4933, 128.54) -> (-139.4933, 128.54)
  line L504 (-139.4933, 128.54) -> (-139.4933, 122.04)
  line L505 (-130.4933, 122.04) -> (-130.4933, 128.54)
  line L506 (-139.4933, 122.04) -> (-130.4933, 122.04)
  line L507 (-138.8933, 127.94) -> (-138.8933, 122.64)
  line L508 (-131.0933, 127.94) -> (-138.8933, 127.94)
  line L509 (-131.0933, 122.64) -> (-131.0933, 127.94)
  line L510 (-148.7467, 122.64) -> (-140.9467, 122.64)
  line L511 (-140.3467, 128.54) -> (-149.3467, 128.54)
  line L512 (-149.3467, 128.54) -> (-149.3467, 122.04)
  line L513 (-140.3467, 122.04) -> (-140.3467, 128.54)
  line L514 (-149.3467, 122.04) -> (-140.3467, 122.04)
  line L515 (-148.7467, 127.94) -> (-148.7467, 122.64)
  line L516 (-140.9467, 127.94) -> (-148.7467, 127.94)
  line L517 (-140.9467, 122.64) -> (-140.9467, 127.94)
  line L518 (-158.6, 122.64) -> (-150.8, 122.64)
  line L519 (-150.2, 128.54) -> (-159.2, 128.54)
  line L520 (-159.2, 128.54) -> (-159.2, 122.04)
  line L521 (-150.2, 122.04) -> (-150.2, 128.54)
  line L522 (-159.2, 122.04) -> (-150.2, 122.04)
  line L523 (-158.6, 127.94) -> (-158.6, 122.64)
  line L524 (-150.8, 127.94) -> (-158.6, 127.94)
  line L525 (-150.8, 122.64) -> (-150.8, 127.94)
  line L526 (-10.8, 112.62) -> (-3, 112.62)
  line L527 (-2.4, 118.52) -> (-11.4, 118.52)
  line L528 (-11.4, 118.52) -> (-11.4, 112.02)
  line L529 (-2.4, 112.02) -> (-2.4, 118.52)
  line L530 (-11.4, 112.02) -> (-2.4, 112.02)
  line L531 (-10.8, 117.92) -> (-10.8, 112.62)
  line L532 (-3, 117.92) -> (-10.8, 117.92)
  line L533 (-3, 112.62) -> (-3, 117.92)
  line L534 (-20.6533, 112.62) -> (-12.8533, 112.62)
  line L535 (-12.2533, 118.52) -> (-21.2533, 118.52)
  line L536 (-21.2533, 118.52) -> (-21.2533, 112.02)
  line L537 (-12.2533, 112.02) -> (-12.2533, 118.52)
  line L538 (-21.2533, 112.02) -> (-12.2533, 112.02)
  line L539 (-20.6533, 117.92) -> (-20.6533, 112.62)
  line L540 (-12.8533, 117.92) -> (-20.6533, 117.92)
  line L541 (-12.8533, 112.62) -> (-12.8533, 117.92)
  line L542 (-30.5067, 112.62) -> (-22.7067, 112.62)
  line L543 (-22.1067, 118.52) -> (-31.1067, 118.52)
  line L544 (-31.1067, 118.52) -> (-31.1067, 112.02)
  line L545 (-22.1067, 112.02) -> (-22.1067, 118.52)
  line L546 (-31.1067, 112.02) -> (-22.1067, 112.02)
  line L547 (-30.5067, 117.92) -> (-30.5067, 112.62)
  line L548 (-22.7067, 117.92) -> (-30.5067, 117.92)
  line L549 (-22.7067, 112.62) -> (-22.7067, 117.92)
  line L550 (-40.36, 112.62) -> (-32.56, 112.62)
  line L551 (-31.96, 118.52) -> (-40.96, 118.52)
  line L552 (-40.96, 118.52) -> (-40.96, 112.02)
  line L553 (-31.96, 112.02) -> (-31.96, 118.52)
  line L554 (-40.96, 112.02) -> (-31.96, 112.02)
  line L555 (-40.36, 117.92) -> (-40.36, 112.62)
  line L556 (-32.56, 117.92) -> (-40.36, 117.92)
  line L557 (-32.56, 112.62) -> (-32.56, 117.92)
  line L558 (-50.2133, 112.62) -> (-42.4133, 112.62)
  line L559 (-41.8133, 118.52) -> (-50.8133, 118.52)
  line L560 (-50.8133, 118.52) -> (-50.8133, 112.02)
  line L561 (-41.8133, 112.02) -> (-41.8133, 118.52)
  line L562 (-50.8133, 112.02) -> (-41.8133, 112.02)
  line L563 (-50.2133, 117.92) -> (-50.2133, 112.62)
  line L564 (-42.4133, 117.92) -> (-50.2133, 117.92)
  line L565 (-42.4133, 112.62) -> (-42.4133, 117.92)
  line L566 (-60.0667, 112.62) -> (-52.2667, 112.62)
  line L567 (-51.6667, 118.52) -> (-60.6667, 118.52)
  line L568 (-60.6667, 118.52) -> (-60.6667, 112.02)
  line L569 (-51.6667, 112.02) -> (-51.6667, 118.52)
  line L570 (-60.6667, 112.02) -> (-51.6667, 112.02)
  line L571 (-60.0667, 117.92) -> (-60.0667, 112.62)
  line L572 (-52.2667, 117.92) -> (-60.0667, 117.92)
  line L573 (-52.2667, 112.62) -> (-52.2667, 117.92)
  line L574 (-69.92, 112.62) -> (-62.12, 112.62)
  line L575 (-61.52, 118.52) -> (-70.52, 118.52)
  line L576 (-70.52, 118.52) -> (-70.52, 112.02)
  line L577 (-61.52, 112.02) -> (-61.52, 118.52)
  line L578 (-70.52, 112.02) -> (-61.52, 112.02)
  line L579 (-69.92, 117.92) -> (-69.92, 112.62)
  line L580 (-62.12, 117.92) -> (-69.92, 117.92)
  line L581 (-62.12, 112.62) -> (-62.12, 117.92)
  line L582 (-79.7733, 112.62) -> (-71.9733, 112.62)
  line L583 (-71.3733, 118.52) -> (-80.3733, 118.52)
  line L584 (-80.3733, 118.52) -> (-80.3733, 112.02)
  line L585 (-71.3733, 112.02) -> (-71.3733, 118.52)
  line L586 (-80.3733, 112.02) -> (-71.3733, 112.02)
  line L587 (-79.7733, 117.92) -> (-79.7733, 112.62)
  line L588 (-71.9733, 117.92) -> (-79.7733, 117.92)
  line L589 (-71.9733, 112.62) -> (-71.9733, 117.92)
  line L590 (-89.6267, 112.62) -> (-81.8267, 112.62)
  line L591 (-81.2267, 118.52) -> (-90.2267, 118.52)
  line L592 (-90.2267, 118.52) -> (-90.2267, 112.02)
  line L593 (-81.2267, 112.02) -> (-81.2267, 118.52)
  line L594 (-90.2267, 112.02) -> (-81.2267, 112.02)
  line L595 (-89.6267, 117.92) -> (-89.6267, 112.62)
  line L596 (-81.8267, 117.92) -> (-89.6267, 117.92)
  line L597 (-81.8267, 112.62) -> (-81.8267, 117.92)
  line L598 (-99.48, 112.62) -> (-91.68, 112.62)
  line L599 (-91.08, 118.52) -> (-100.08, 118.52)
  line L600 (-100.08, 118.52) -> (-100.08, 112.02)
  line L601 (-91.08, 112.02) -> (-91.08, 118.52)
  line L602 (-100.08, 112.02) -> (-91.08, 112.02)
  line L603 (-99.48, 117.92) -> (-99.48, 112.62)
  line L604 (-91.68, 117.92) -> (-99.48, 117.92)
  line L605 (-91.68, 112.62) -> (-91.68, 117.92)
  line L606 (-109.3333, 112.62) -> (-101.5333, 112.62)
  line L607 (-100.9333, 118.52) -> (-109.9333, 118.52)
  line L608 (-109.9333, 118.52) -> (-109.9333, 112.02)
  line L609 (-100.9333, 112.02) -> (-100.9333, 118.52)
  line L610 (-109.9333, 112.02) -> (-100.9333, 112.02)
  line L611 (-109.3333, 117.92) -> (-109.3333, 112.62)
  line L612 (-101.5333, 117.92) -> (-109.3333, 117.92)
  line L613 (-101.5333, 112.62) -> (-101.5333, 117.92)
  line L614 (-119.1867, 112.62) -> (-111.3867, 112.62)
  line L615 (-110.7867, 118.52) -> (-119.7867, 118.52)
  line L616 (-119.7867, 118.52) -> (-119.7867, 112.02)
  line L617 (-110.7867, 112.02) -> (-110.7867, 118.52)
  line L618 (-119.7867, 112.02) -> (-110.7867, 112.02)
  line L619 (-119.1867, 117.92) -> (-119.1867, 112.62)
  line L620 (-111.3867, 117.92) -> (-119.1867, 117.92)
  line L621 (-111.3867, 112.62) -> (-111.3867, 117.92)
  line L622 (-129.04, 112.62) -> (-121.24, 112.62)
  line L623 (-120.64, 118.52) -> (-129.64, 118.52)
  line L624 (-129.64, 118.52) -> (-129.64, 112.02)
  line L625 (-120.64, 112.02) -> (-120.64, 118.52)
  line L626 (-129.64, 112.02) -> (-120.64, 112.02)
  line L627 (-129.04, 117.92) -> (-129.04, 112.62)
  line L628 (-121.24, 117.92) -> (-129.04, 117.92)
  line L629 (-121.24, 112.62) -> (-121.24, 117.92)
  line L630 (-138.8933, 112.62) -> (-131.0933, 112.62)
  line L631 (-130.4933, 118.52) -> (-139.4933, 118.52)
  line L632 (-139.4933, 118.52) -> (-139.4933, 112.02)
  line L633 (-130.4933, 112.02) -> (-130.4933, 118.52)
  line L634 (-139.4933, 112.02) -> (-130.4933, 112.02)
  line L635 (-138.8933, 117.92) -> (-138.8933, 112.62)
  line L636 (-131.0933, 117.92) -> (-138.8933, 117.92)
  line L637 (-131.0933, 112.62) -> (-131.0933, 117.92)
  line L638 (-148.7467, 112.62) -> (-140.9467, 112.62)